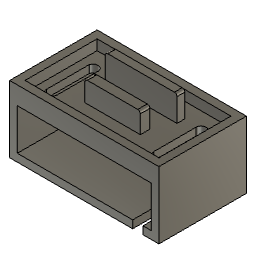
cable_box (Autodesk Fusion 360 design; units mm, degrees)
Autodesk Fusion 360 part; units mm, degrees
sketch "bottom" plane through (0, 0, 0) normal (0, 0, 1) x (1, 0, 0)
  line L0 (0, 0) -> (-290, 0)
  line L1 (-290, 0) -> (-290, 170)
  line L2 (-290, 170) -> (0, 170)
  line L3 (0, 170) -> (0, 0)
  dimension "d41" = 290
  dimension "d42" = 170
  constraint horizontal L0
  constraint vertical L1
  constraint horizontal L2
  constraint vertical L3
  constraint coincident L0.start L3.end
  measures "d41" distance of L1.end L2.end
  measures "d42" distance of L0.end L1.end
extrude "Extrude1" add sketch "bottom" along normal blind 110
shell "Shell1" thickness 15 removed faces 1 at (-96.6667, 0, 36.6667)
sketch "Sketch5" plane through (0, 0, 15) normal (0, 0, 1) x (-1, 0, 0)
  line L0 (15, -155) -> (275, -155)
  line L1 (275, -155) -> (275, 0)
  line L2 (275, 0) -> (15, 0)
  line L3 (15, 0) -> (15, -155)
  arc A0 (91.5155, -197.8612) -> (90.4492, -197.9194) centre (90.9821, -197.8846) ccw
sketch "general cable" plane through (0, 0, 0) normal (0, 0, 1) x (1, 0, 0)
  line L0 (-30.8887, -0.5052) -> (-30.8887, 139.4948)
  arc A0 (-30.8887, 139.4948) -> (-50.8736, 139.4948) centre (-40.8811, 139.4948) ccw
  line L1 (-50.8736, 139.4948) -> (-50.8736, -0.4766)
  line L2 (-50.8736, -0.4766) -> (-30.8887, -0.5052)
  dimension "d5" = 140
  constraint vertical L0
  constraint tangent L0 A0
  constraint tangent A0 L1
  constraint vertical L1
  measures "d5" distance of L0.start L0.end
extrude "Extrude2" cut sketch "general cable" along normal blind 20
sketch "Sketch7" plane through (0, 0, 110) normal (0, 0, 1) x (-1, 0, 0)
  line L0 (0, -170) -> (290, -170)
  line L1 (290, -170) -> (290, 0)
  line L2 (290, 0) -> (0, 0)
  line L3 (0, 0) -> (0, -170)
  line L4 (0, 0) -> (290, 0)
  line L5 (290, 0) -> (290, -170)
  line L6 (290, -170) -> (0, -170)
  line L7 (0, -170) -> (0, 0)
  constraint horizontal L4
  constraint vertical L5
  constraint horizontal L6
  constraint vertical L7
  constraint coincident L0.end L1.start
  constraint coincident L2.end L3.start
extrude "Extrude3" add sketch "Sketch7" along normal blind 20
shell "Shell2" thickness 15 removed faces 1 at (-96.6667, 56.6667, 130)
sketch "cable2" plane through (0, 0, 110) normal (0, 0, 1) x (-1, 0, 0)
  line L0 (15, -155) -> (275, -155)
  line L1 (275, -155) -> (275, -15)
  line L2 (275, -15) -> (15, -15)
  line L3 (15, -15) -> (15, -155)
  line L4 (30.602, -40.8015) -> (30.602, -122.3767)
  arc A0 (30.602, -122.3767) -> (50.2207, -122.3767) centre (40.4114, -122.3767) ccw
  line L5 (50.2207, -122.3767) -> (50.2207, -40.4606)
  arc A1 (50.2207, -40.4606) -> (30.602, -40.8015) centre (40.4084, -40.4606) ccw
  constraint vertical L4
  constraint tangent L4 A0
  constraint tangent A0 L5
  constraint parallel L4 L5
  constraint tangent L5 A1
extrude "Extrude4" cut sketch "cable2" against normal blind 20 contours L4 A0 L5 A1
sketch "cable" plane through (0, 0, 110) normal (0, 0, 1) x (-1, 0, 0)
  line L0 (30.602, -122.3767) -> (30.602, -40.8015)
  arc A0 (50.2207, -40.4606) -> (30.602, -40.8015) centre (40.4084, -40.4606) ccw
  line L1 (50.2207, -40.4606) -> (50.2207, -122.3767)
  arc A1 (30.602, -122.3767) -> (50.2207, -122.3767) centre (40.4114, -122.3767) ccw
  line L2 (15, -155) -> (275, -155)
  line L3 (275, -155) -> (275, -15)
  line L4 (275, -15) -> (15, -15)
  line L5 (15, -15) -> (15, -155)
  line L6 (259.2195, -123.7608) -> (259.2195, -41.0341)
  arc A2 (259.2195, -41.0341) -> (239.4378, -41.0341) centre (249.3287, -41.0341) ccw
  line L7 (239.4378, -41.0341) -> (239.4378, -121.3669)
  arc A3 (239.4378, -121.3669) -> (259.2195, -123.7608) centre (249.4735, -121.3669) ccw
  constraint parallel L3 L6
  constraint tangent L6 A2
  constraint tangent A2 L7
  constraint parallel L6 L7
  constraint tangent L7 A3
extrude "Extrude5" cut sketch "cable" against normal blind 20 contours L6 A2 L7 A3
sketch "wedge big" plane through (0, 0, 110) normal (0, 0, 1) x (-1, 0, 0)
  line L0 (30.602, -122.3767) -> (30.602, -40.8015)
  arc A0 (50.2207, -40.4606) -> (30.602, -40.8015) centre (40.4084, -40.4606) ccw
  line L1 (50.2207, -40.4606) -> (50.2207, -122.3767)
  arc A1 (30.602, -122.3767) -> (50.2207, -122.3767) centre (40.4114, -122.3767) ccw
  line L2 (15, -155) -> (275, -155)
  line L3 (275, -155) -> (275, -15)
  line L4 (275, -15) -> (15, -15)
  line L5 (15, -15) -> (15, -155)
  line L6 (214.6228, -110.316) -> (75.1991, -110.316)
  line L7 (75.1991, -110.316) -> (75.1991, -125.4165)
  line L8 (75.1991, -125.4165) -> (214.6228, -125.4165)
  line L9 (214.6228, -125.4165) -> (214.6228, -110.316)
  line L10 (259.2195, -41.0341) -> (259.2195, -123.7608)
  arc A2 (239.4378, -121.3669) -> (259.2195, -123.7608) centre (249.4735, -121.3669) ccw
  line L11 (239.4378, -121.3669) -> (239.4378, -41.0341)
  arc A3 (259.2195, -41.0341) -> (239.4378, -41.0341) centre (249.3287, -41.0341) ccw
  constraint horizontal L6
  constraint vertical L7
  constraint horizontal L8
  constraint vertical L9
extrude "Extrude6" add sketch "wedge big" along normal blind 40 contours L6 L7 L8 L9
sketch "wedge small" plane through (0, 0, 110) normal (0, 0, 1) x (-1, 0, 0)
  line L0 (30.602, -122.3767) -> (30.602, -40.8015)
  arc A0 (50.2207, -40.4606) -> (30.602, -40.8015) centre (40.4084, -40.4606) ccw
  line L1 (50.2207, -40.4606) -> (50.2207, -122.3767)
  arc A1 (30.602, -122.3767) -> (50.2207, -122.3767) centre (40.4114, -122.3767) ccw
  line L2 (15, -155) -> (275, -155)
  line L3 (275, -155) -> (275, -15)
  line L4 (275, -15) -> (15, -15)
  line L5 (15, -15) -> (15, -155)
  line L6 (199.6701, -74.1952) -> (91.7665, -74.1952)
  line L7 (91.7665, -74.1952) -> (91.7665, -55.7304)
  line L8 (91.7665, -55.7304) -> (199.6701, -55.7304)
  line L9 (199.6701, -55.7304) -> (199.6701, -74.1952)
  line L10 (214.6228, -125.4165) -> (75.1991, -125.4165)
  line L11 (75.1991, -125.4165) -> (75.1991, -110.316)
  line L12 (75.1991, -110.316) -> (214.6228, -110.316)
  line L13 (214.6228, -110.316) -> (214.6228, -125.4165)
  line L14 (259.2195, -41.0341) -> (259.2195, -123.7608)
  arc A2 (239.4378, -121.3669) -> (259.2195, -123.7608) centre (249.4735, -121.3669) ccw
  line L15 (239.4378, -121.3669) -> (239.4378, -41.0341)
  arc A3 (259.2195, -41.0341) -> (239.4378, -41.0341) centre (249.3287, -41.0341) ccw
  constraint horizontal L6
  constraint vertical L7
  constraint horizontal L8
  constraint vertical L9
extrude "Extrude7" add sketch "wedge small" along normal blind 40 contours L6 L7 L8 L9
extrude "Extrude8" add 1 faces at (-121.6737, 120.383, 150) along direction (0, 0, 1) blind 30
extrude "Extrude9" cut 1 faces at (-121.6737, 120.383, 180) along direction (0, 0, -1) blind 20
fillet "Fillet7" radius 5 2 edges at (-214.6228, 117.8662, 160) (-75.1991, 117.8662, 160)
fillet "Fillet8" radius 5 2 edges at (-199.6701, 64.9628, 150) (-91.7665, 64.9628, 150)
fillet "Fillet9" [rolled back] radius 10
